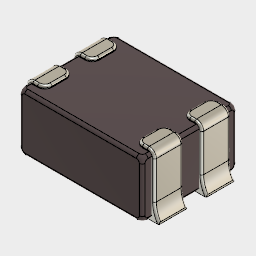
capar2_1013 (Autodesk Fusion 360 design; units mm, degrees)
Autodesk Fusion 360 part; units mm, degrees
ref_plane "WorkPlane4" through (0, 0, 0.02) normal (0, 0, 1) x (1, 0, 0)
sketch "Sketch5" plane through (0, 0, 0.02) normal (0, 0, 1) x (1, 0, 0)
  line L0 (0.65, -0.5) -> (-0.65, -0.5)
  line L1 (-0.65, -0.5) -> (-0.65, 0.5)
  line L2 (-0.65, 0.5) -> (0.65, 0.5)
  line L3 (0.65, 0.5) -> (0.65, -0.5)
  line L4 (0.65, -0.5) -> (-0.65, 0.5) construction
  line L5 (-0.65, -0.5) -> (0.65, 0.5) construction
  dimension "d38" = 1.3
  dimension "d39" = 1
  measures "d38" distance of L1.end L2.end
  measures "d39" distance of L0.end L1.end
extrude "Extrude4" add sketch "Sketch5" along normal blind 0.6 makes body 1
fillet "Fillet6" radius 0.03 12 edges at (-0.65, -0.5, 0.32) (-0.65, 0, 0.62) (0, 0.5, 0.62) (0, -0.5, 0.62) (-0.65, 0.5, 0.32) (-0.65, 0, 0.02) (0, -0.5, 0.02) (0, 0.5, 0.02) (0.65, 0, 0.62) (0.65, 0.5, 0.32) (0.65, -0.5, 0.32) (0.65, 0, 0.02) on bodies 1
sketch "Sketch7" plane through (0, 0, 0.02) normal (0, 0, 1) x (1, 0, 0)
  line L0 (-0.725, 0.4) -> (-0.275, 0.4)
  line L1 (-0.275, 0.4) -> (-0.275, 0.1)
  line L2 (-0.275, 0.1) -> (-0.725, 0.1)
  line L3 (-0.725, 0.1) -> (-0.725, 0.4)
  line L4 (0, 0) -> (-0.5, 0) construction
  line L5 (0, 0) -> (0, 0.4016) construction
  line L6 (-0.275, -0.4) -> (-0.275, -0.1)
  line L7 (-0.275, -0.1) -> (-0.725, -0.1)
  line L8 (-0.725, -0.1) -> (-0.725, -0.4)
  line L9 (-0.725, -0.4) -> (-0.275, -0.4)
  line L10 (0.725, 0.4) -> (0.275, 0.4)
  line L11 (0.275, 0.4) -> (0.275, 0.1)
  line L12 (0.275, 0.1) -> (0.725, 0.1)
  line L13 (0.725, 0.1) -> (0.725, 0.4)
  line L14 (0.725, -0.4) -> (0.275, -0.4)
  line L15 (0.275, -0.4) -> (0.275, -0.1)
  line L16 (0.725, -0.1) -> (0.725, -0.4)
  line L17 (0.275, -0.1) -> (0.725, -0.1)
  line L18 (-0.68, 0.4) -> (-0.68, 0.1)
  line L19 (-0.68, -0.1) -> (-0.68, -0.4)
  line L20 (-0.62, 0.4) -> (-0.62, 0.1)
  line L21 (-0.62, -0.1) -> (-0.62, -0.4)
  line L22 (0.68, 0.4) -> (0.68, 0.1)
  line L23 (0.62, 0.4) -> (0.62, 0.1)
  line L24 (0.68, -0.1) -> (0.68, -0.4)
  line L25 (0.62, -0.1) -> (0.62, -0.4)
  dimension "d41" = 0.45
  dimension "d42" = 0.3
  dimension "d43" = 1
  dimension "d44" = 0.5
  dimension "d45" = 0.62
  dimension "d46" = 0.06
  measures "d41" distance of L0.start L0.end
  measures "d42" distance of L0.start L2.end
  measures "d43" distance of L1 L13
  measures "d44" distance of L2 L9
  measures "d45" distance of L4.start L20
  measures "d46" distance of L18 L20
extrude "Extrude8" add sketch "Sketch7" against normal blind 0.02 separate body makes body 2 at (0.425, 0.3, 0.02) makes body 3 at (0.575, -0.3, 0.02) makes body 4 at (-0.575, 0.3, 0.02) makes body 5 at (-0.425, -0.3, 0.02)
extrude "Extrude9" add sketch "Sketch7" along normal blind 0.6 contours L0 L2 L18 L20 | L7 L9 L19 L21 | L10 L12 L22 L23 | L14 L17 L24 L25 bodies 2 3 4 5
sketch "Sketch6" plane through (0, 0, 0.62) normal (0, 0, 1) x (-1, 0, 0)
  line L0 (0, 0) -> (0.35, 0) construction
  line L1 (0, 0) -> (0, -0.4804) construction
  line L2 (0.68, 0.1) -> (0.48, 0.1)
  line L3 (0.48, 0.1) -> (0.48, 0.4)
  line L4 (0.48, 0.4) -> (0.68, 0.4)
  line L5 (0.68, 0.4) -> (0.68, 0.1)
  line L6 (0.68, -0.4) -> (0.68, -0.1)
  line L7 (0.68, -0.1) -> (0.48, -0.1)
  line L8 (0.48, -0.1) -> (0.48, -0.4)
  line L9 (0.48, -0.4) -> (0.68, -0.4)
  line L10 (-0.48, -0.1) -> (-0.48, -0.4)
  line L11 (-0.48, -0.4) -> (-0.68, -0.4)
  line L12 (-0.68, -0.4) -> (-0.68, -0.1)
  line L13 (-0.68, -0.1) -> (-0.48, -0.1)
  line L14 (-0.68, 0.4) -> (-0.68, 0.1)
  line L15 (-0.68, 0.1) -> (-0.48, 0.1)
  line L16 (-0.48, 0.4) -> (-0.68, 0.4)
  line L17 (-0.48, 0.1) -> (-0.48, 0.4)
  line L18 (0.68, 0.1) -> (0.68, 0.4)
  line L19 (0.68, 0.4) -> (0.62, 0.4)
  line L20 (0.62, 0.1) -> (0.68, 0.1)
  point P0 (0.68, 0.4)
  dimension "d51" = 0.2
  measures "d51" distance of L3 L5
extrude "Extrude7" add sketch "Sketch6" along normal blind 0.03 bodies 2 3 4 5
fillet "Fillet5" radius 0.3 4 edges at (0.68, 0.25, 0.02) (0.68, -0.25, 0.02) (-0.68, 0.25, 0.02) (-0.68, -0.25, 0.02) on bodies 2 3 4 5
fillet "Fillet5" radius 0.075 12 edges at (0.48, 0.1, 0.635) (0.48, 0.4, 0.635) (0.68, 0.25, 0.65) (0.68, -0.25, 0.65) (0.48, -0.4, 0.635) (0.48, -0.1, 0.635) (-0.68, 0.25, 0.65) (-0.48, 0.1, 0.635) (-0.48, 0.4, 0.635) (-0.48, -0.4, 0.635) (-0.48, -0.1, 0.635) (-0.68, -0.25, 0.65) on bodies 2 3 4 5
fillet "Fillet7" radius 0.02 44 edges at (0.6915, 0.1, 0.0959) (0.68, 0.1, 0.3765) (0.658, 0.1, 0.628) (0.58, 0.1, 0.65) (0.502, 0.122, 0.65) (0.48, 0.25, 0.65) (0.502, 0.378, 0.65) (0.58, 0.4, 0.65) (0.658, 0.4, 0.628) (0.68, 0.4, 0.3765) (0.6915, 0.4, 0.0959) (0.6915, -0.4, 0.0959) (0.68, -0.4, 0.3765) (0.658, -0.4, 0.628) (0.58, -0.4, 0.65) (0.502, -0.378, 0.65) (0.48, -0.25, 0.65) (0.502, -0.122, 0.65) (0.58, -0.1, 0.65) (0.658, -0.1, 0.628) (0.68, -0.1, 0.3765) (0.6915, -0.1, 0.0959) (-0.6915, 0.4, 0.0959) (-0.68, 0.4, 0.3765) (-0.658, 0.4, 0.628) (-0.58, 0.4, 0.65) (-0.502, 0.378, 0.65) (-0.48, 0.25, 0.65) (-0.502, 0.122, 0.65) (-0.58, 0.1, 0.65) (-0.658, 0.1, 0.628) (-0.68, 0.1, 0.3765) (-0.6915, 0.1, 0.0959) (-0.6915, -0.1, 0.0959) (-0.68, -0.1, 0.3765) (-0.658, -0.1, 0.628) (-0.58, -0.1, 0.65) (-0.502, -0.122, 0.65) (-0.48, -0.25, 0.65) (-0.502, -0.378, 0.65) (-0.58, -0.4, 0.65) (-0.658, -0.4, 0.628) (-0.68, -0.4, 0.3765) (-0.6915, -0.4, 0.0959) on bodies 2 3 4 5
equation "capar2_1310_height = 0.6 mm"
equation "capar2_1310_width = 1 mm"
equation "capar2_1310_length = 1.3 mm"
equation "capar2_1310_tin_len = 0.2 mm"
equation "capar2_1310_tin_thick_axial = 0.06 mm"
equation "capar2_1310_land_width_spacing = 0.5 mm"
equation "capar2_1310_land_width = 0.3 mm"
equation "capar2_1310_land_length = 0.45 mm"
equation "capar2_1310_above_board = 0.02 mm"
equation "d6 = capar2_1310_above_board"
equation "capar2_1310_land_length_spacing = 1 mm"
equation "d17 = capar2_1310_height"
equation "d26 = capar2_1310_tin_thick_axial / 2"
equation "d38 = capar2_1310_length"
equation "d39 = capar2_1310_width"
equation "d41 = capar2_1310_land_length"
equation "d42 = capar2_1310_land_width"
equation "d43 = capar2_1310_land_length_spacing"
equation "d44 = capar2_1310_land_width_spacing"
equation "d45 = capar2_1310_length / 2 - capar2_1310_tin_thick_axial / 2"
equation "d46 = capar2_1310_tin_thick_axial"
equation "d47 = -capar2_1310_above_board"
equation "d49 = capar2_1310_height"
equation "d51 = capar2_1310_tin_len"
equation "d52 = capar2_1310_height / 2"
